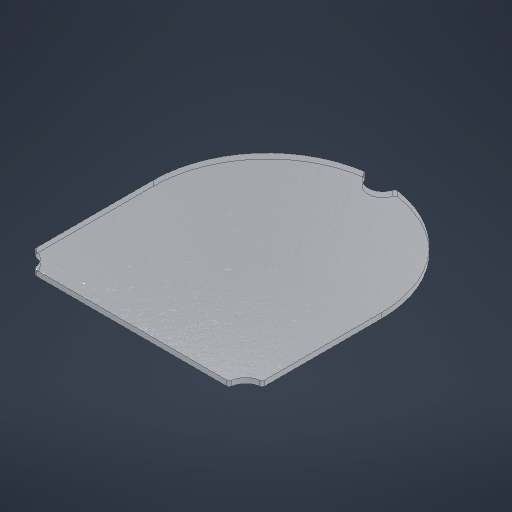
# Autodesk Inventor part: acrylic_lens
Saved by Autodesk Inventor 2026.2 (Build 302298000, 298)
## iProperties
Created: 2026-04-07
Part Number: acrylic_lens
Material: Acrylic, Clear
Document SubType Name: Modeling
Designer: Tathagata Sikdar
Density: 1.19 g/cm^3
Appearance: Transparent - Clear
Author: Tathagata Sikdar
Autodesk Inventor part; units mm, degrees
ref_plane "YZ Plane" through (0, 0, 0) normal (1, 0, 0) x (0, 1, 0)
ref_plane "XZ Plane" through (0, 0, 0) normal (0, 1, 0) x (-1, 0, 0)
ref_plane "Work Plane1" through (77.4141, 48.0807, 96.7749) normal (0, 1, 0) x (-1, 0, 0)
sketch "Sketch1" plane through (77.4141, 48.0807, 96.7749) normal (0, 1, 0) x (-1, 0, 0)
  arc A0 (-12.9956, -95.0875) -> (-10.7767, -93.6645) centre (-12.6982, -93.1097) ccw projected
  arc A1 (10.7767, -93.6645) -> (-10.7767, -93.6645) centre (0, -96.776) ccw projected
  arc A2 (10.7767, -93.6645) -> (12.9956, -95.0875) centre (12.6982, -93.1097) ccw projected
  arc A3 (12.9956, -95.0875) -> (32.2927, -89.8741) centre (0, -8.6647) ccw projected
  line L0 (32.2927, -89.8741) -> (32.2927, -92.3799) projected
  arc A4 (32.2927, -92.3799) -> (39.7927, -92.3799) centre (36.0427, -92.3799) ccw projected
  line L1 (39.7927, -92.3799) -> (39.7927, -86.4742) projected
  arc A5 (39.7927, -86.4742) -> (87.075, -16.1299) centre (0, -8.6647) ccw projected
  line L2 (87.075, -16.1299) -> (91.0687, -16.1299) projected
  arc A6 (91.0687, -16.1299) -> (91.0687, -8.6299) centre (91.0687, -12.3799) ccw projected
  line L3 (91.0687, -8.6299) -> (87.3944, -8.6299) projected
  line L4 (87.3944, -8.6299) -> (87.3944, 63.8701) projected
  line L5 (87.3944, 63.8701) -> (91.1444, 63.8701) projected
  arc A7 (91.1444, 63.8701) -> (91.1444, 71.3701) centre (91.1444, 67.6201) ccw projected
  line L6 (91.1444, 71.3701) -> (87.3944, 71.3701) projected
  line L7 (87.3944, 71.3701) -> (87.3944, 80.7566) projected
  arc A8 (87.3944, 80.7566) -> (85.666, 82.738) centre (85.3944, 80.7566) ccw projected
  arc A9 (74.7844, 93.6197) -> (85.666, 82.738) centre (87.3944, 95.3481) ccw projected
  arc A10 (74.7844, 93.6197) -> (72.8029, 95.3481) centre (72.8029, 93.3481) ccw projected
  line L8 (72.8029, 95.3481) -> (-72.8029, 95.3481) projected
  arc A11 (-72.8029, 95.3481) -> (-74.7844, 93.6197) centre (-72.8029, 93.3481) ccw projected
  arc A12 (-85.666, 82.738) -> (-74.7844, 93.6197) centre (-87.3944, 95.3481) ccw projected
  arc A13 (-85.666, 82.738) -> (-87.3944, 80.7566) centre (-85.3944, 80.7566) ccw projected
  line L9 (-87.3944, 80.7566) -> (-87.3944, 71.3701) projected
  line L10 (-87.3944, 71.3701) -> (-91.1444, 71.3701) projected
  arc A14 (-91.1444, 71.3701) -> (-91.1444, 63.8701) centre (-91.1444, 67.6201) ccw projected
  line L11 (-91.1444, 63.8701) -> (-87.3944, 63.8701) projected
  line L12 (-87.3944, 63.8701) -> (-87.3944, -8.6299) projected
  line L13 (-87.3944, -8.6299) -> (-91.1444, -8.6299) projected
  arc A15 (-91.1444, -8.6299) -> (-91.1444, -16.1299) centre (-91.1444, -12.3799) ccw projected
  line L14 (-91.1444, -16.1299) -> (-87.075, -16.1299) projected
  arc A16 (-87.075, -16.1299) -> (-39.7927, -86.4742) centre (0, -8.6647) ccw projected
  line L15 (-39.7927, -86.4742) -> (-39.7927, -92.3799) projected
  arc A17 (-39.7927, -92.3799) -> (-32.2927, -92.3799) centre (-36.0427, -92.3799) ccw projected
  line L16 (-32.2927, -92.3799) -> (-32.2927, -89.8741) projected
  arc A18 (-32.2927, -89.8741) -> (-12.9956, -95.0875) centre (0, -8.6647) ccw projected
  circle A19 centre (-36.0427, -92.3799) radius 1.85 projected
  circle A20 centre (91.1444, 67.6201) radius 1.85 projected
  circle A21 centre (36.0427, -92.3799) radius 1.85 projected
  circle A22 centre (-91.1444, 67.6201) radius 1.85 projected
  circle A23 centre (-91.1444, -12.3799) radius 1.85 projected
  circle A24 centre (91.0687, -12.3799) radius 1.85 projected
  arc A25 (85.9744, 79.5665) -> (84.398, 81.5211) centre (83.9744, 79.5665) ccw projected
  line L17 (85.9744, 79.5665) -> (85.9744, -8.6647) projected
  arc A26 (13.9862, -93.4939) -> (85.9744, -8.6647) centre (0, -8.6647) ccw projected
  arc A27 (11.7942, -92.2386) -> (13.9862, -93.4939) centre (13.6608, -91.5205) ccw projected
  arc A28 (11.7942, -92.2386) -> (-11.7942, -92.2386) centre (0, -96.776) ccw projected
  arc A29 (-13.9862, -93.4939) -> (-11.7942, -92.2386) centre (-13.6608, -91.5205) ccw projected
  arc A30 (-85.9744, -8.6647) -> (-13.9862, -93.4939) centre (0, -8.6647) ccw projected
  line L18 (-85.9744, -8.6647) -> (-85.9744, 79.5665) projected
  arc A31 (-84.398, 81.5211) -> (-85.9744, 79.5665) centre (-83.9744, 79.5665) ccw projected
  arc A32 (-84.398, 81.5211) -> (-73.5675, 92.3516) centre (-87.3944, 95.3481) ccw projected
  arc A33 (-71.6128, 93.9281) -> (-73.5675, 92.3516) centre (-71.6128, 91.9281) ccw projected
  line L19 (-71.6128, 93.9281) -> (71.6128, 93.9281) projected
  arc A34 (73.5675, 92.3516) -> (71.6128, 93.9281) centre (71.6128, 91.9281) ccw projected
  arc A35 (73.5675, 92.3516) -> (84.398, 81.5211) centre (87.3944, 95.3481) ccw projected
  arc A36 (32.2927, -89.8741) -> (39.7927, -86.4742) centre (0, -8.6647) ccw
  arc A37 (-39.7927, -86.4742) -> (-32.2927, -89.8741) centre (0, -8.6647) ccw
  arc A38 (-87.3944, -8.6299) -> (-87.075, -16.1299) centre (0, -8.6647) ccw
  line L20 (-87.3944, 71.3701) -> (-87.3944, 63.8701)
  line L21 (87.3944, 71.3701) -> (87.3944, 63.8701)
  arc A39 (87.075, -16.1299) -> (87.3944, -8.6299) centre (0, -8.6647) ccw
  point P0 (77.4141, -96.7749)
  constraints: 8 point on circle, 4 centre point, 4 concentric, 4 end point, 1 parallel, 1 vertical
extrude "Extrusion1" add sketch "Sketch1" along normal blind 4 contours A18 A37 A16 A38 L12 L20 L9 A13 A12 A11 L8 A10 A9 A8 L7 L21 L4 A39 A5 A36 A3 A2 A1 A0 | L17 A26 A27 A28 A29 A30 L18 A31 A32 A33 L19 A34 A35 A25
body "Solid1"
